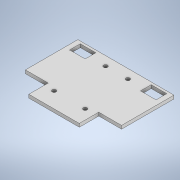
# Autodesk Inventor part: PlacaInferior
Saved by Autodesk Inventor 2021 (Build 250183000, 183)
## iProperties
Created: 2021-10-29
Part Number: PlacaInferior
Material: Genérico
Document SubType Name: Chapa
Designer: Juan Camilo
Density: 1 g/cm^3
Sheet Metal Rule: Por defecto_mm
Appearance: Valor por defecto
Author: Juan Camilo
Autodesk Inventor part; units mm, degrees
ref_plane "YZ Plane" through (0, 0, 0) normal (1, 0, 0) x (0, 1, 0)
ref_plane "XZ Plane" through (0, 0, 0) normal (0, 1, 0) x (-1, 0, 0)
ref_plane "XY Plane" through (0, 0, 0) normal (0, 0, 1) x (1, 0, 0)
sketch "Boceto1" plane through (0, 0, 0) normal (0, 1, 0) x (-1, 0, 0)
  line L0 (-71.0974, 28.13) -> (-71.0974, -25.87)
  line L1 (-71.0974, -25.87) -> (27.9026, -25.87)
  line L2 (27.9026, -25.87) -> (27.9026, 28.13)
  line L3 (4.4026, 48.13) -> (-47.5974, 48.13)
  line L4 (-47.5974, 48.13) -> (-47.5974, 28.13)
  line L5 (4.4026, 28.13) -> (4.4026, 48.13)
  line L6 (27.9026, 28.13) -> (4.4026, 28.13)
  line L7 (-47.5974, 28.13) -> (-71.0974, 28.13)
  circle A0 centre (-5.5974, 32.13) radius 2
  line L8 (-21.5974, 48.13) -> (-21.5974, -25.87)
  circle A1 centre (-37.5974, 32.13) radius 2
  line L9 (22.9026, -12.37) -> (6.9026, -12.37)
  line L10 (6.9026, -12.37) -> (6.9026, -23.37)
  line L11 (6.9026, -23.37) -> (22.9026, -23.37)
  line L12 (22.9026, -23.37) -> (22.9026, -12.37)
  line L13 (-66.0974, -12.37) -> (-50.0974, -12.37)
  line L14 (-50.0974, -12.37) -> (-50.0974, -23.37)
  line L15 (-50.0974, -23.37) -> (-66.0974, -23.37)
  line L16 (-66.0974, -23.37) -> (-66.0974, -12.37)
  circle A2 centre (-10.0974, -16.37) radius 2
  circle A3 centre (-33.0974, -16.37) radius 2
  point P0 (0, 0)
  dimension "d0" = 54
  dimension "d1" = 99
  dimension "d2" = 20
  dimension "d3" = 52
  dimension "d4" = 23.5
  dimension "d5" = 23.5
  dimension "d6" = 4
  dimension "d7" = 16
  dimension "d8" = 10
  dimension "d9" = 2.5
  dimension "d10" = 5
  dimension "d11" = 11
  dimension "d12" = 16
  dimension "d13" = 4
  dimension "d15" = 9.5
  dimension "d18" = 36
  dimension "d19" = 17
  constraints: 34 end point, 6 parallel, 6 symmetric about line, 4 centre point, 4 horizontal, 4 perpendicular, 2 midpoint, 2 other
  measures "d0" distance of L1.end L2.end
  measures "d1" distance of L2.end L0.start
  measures "d2" distance of L5.start L3.start
  measures "d3" distance of L3.start L3.end
  measures "d4" distance from line of L5 L2.end
  measures "d5" distance from line of L0.start L4
  measures "d6" diameter of A0
  measures "d7" distance from line of A0.centre L3
  measures "d8" distance from line of L5 A0.centre
  measures "d9" distance between parallel lines of L1 L11
  measures "d10" distance between parallel lines of L12 L2
  measures "d11" distance of L9.end L10.end
  measures "d12" distance of L9.start L9.end
  measures "d13" diameter of A2
  measures "d15" distance from line of L1 A2.centre
  measures "d18" distance edge to line of A2 L2
  measures "d19" distance from line of A2.centre L10
extrude "Extrusión1" add sketch "Boceto1" along normal blind 3.4
equation "\"Radio_pliegue\" = Grosor"
equation "\"Anchura_desahogo_plegado\" = Grosor"
equation "\"Profundidad_desahogo_plegado\" = 0.5 * Grosor"
equation "\"Tamaño_destalonado\" = 4 * Grosor"
equation "\"Remanente_mínimo\" = 2 * Grosor"
equation "\"Radiodetransición\" = Radio_pliegue"
equation "\"Tamaño_de_radio_de_Jacobi\" = Radio_pliegue"
equation "\"TamañoSeparación\" = Grosor"
equation "\"Grosor\" = 0.5"
